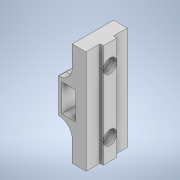
# Autodesk Inventor part: Mount Female
Saved by Autodesk Inventor 2020 (Build 240168000, 168)
## iProperties
Created: 2020-01-14
Part Number: Mount Female
Material: Generic
Document SubType Name: Modeling
Designer: maple
Density: 1 g/cm^3
Appearance: Default
Author: maple
Autodesk Inventor part; units mm, degrees
ref_plane "YZ Plane" through (0, 0, 0) normal (1, 0, 0) x (0, 1, 0)
ref_plane "XZ Plane" through (0, 0, 0) normal (0, 1, 0) x (-1, 0, 0)
ref_plane "XY Plane" through (0, 0, 0) normal (0, 0, 1) x (1, 0, 0)
sketch "Sketch1" plane through (0, 0, 0) normal (0, 1, 0) x (-1, 0, 0)
  line L0 (0, 0) -> (-5.08, 0)
  line L1 (-5.08, 0) -> (-5.08, -15.24)
  line L2 (-5.08, -15.24) -> (0, -15.24)
  line L3 (0, -15.24) -> (0, 0)
  line L4 (-5.08, -7.62) -> (-5.08, -5.08)
  line L5 (-5.08, -5.08) -> (-8.89, -5.08)
  line L6 (-8.89, -5.08) -> (-8.89, -2.54)
  line L7 (-8.89, -5.08) -> (-11.43, -5.08)
  line L8 (-11.43, -5.08) -> (-11.43, -10.16)
  line L9 (-11.43, -10.16) -> (-5.08, -10.16)
  line L10 (-8.89, -10.16) -> (-8.89, -12.7)
  line L11 (-8.89, -12.7) -> (-11.43, -10.16)
  line L12 (-8.89, -2.54) -> (-11.43, -5.08)
  dimension "d0" = 5.08
  dimension "d1" = 15.24
  dimension "d2" = 2.54
  dimension "d3" = 3.81
  dimension "d4" = 2.54
  dimension "d5" = 2.54
  dimension "d6" = 5.08
  dimension "d7" = 2.54
  constraints: 26 end point, 5 perpendicular, 3 point on line, 2 horizontal, 2 parallel, 2 vertical, 1 midpoint
  measures "d0" distance of L2.end L1.end
  measures "d1" distance of L1.end L0.end
  measures "d2" distance of L4.start L4.end
  measures "d3" distance of L4.end L5.end
  measures "d4" distance of L5.end L6.end
  measures "d5" distance of L5.end L7.end
  measures "d6" distance of L7.end L8.end
  measures "d7" distance of L10.start L10.end
extrude "Extrusion1" add sketch "Sketch1" along normal blind 38.1
sketch "Sketch2" plane through (0, 0, -15.24) normal (-1, 0, 0) x (0, 0, 1)
  line L0 (10.16, 0) -> (5.08, 0) projected
  line L1 (7.62, 0) -> (7.62, 7.62)
  line L2 (10.16, 38.1) -> (5.08, 38.1) projected
  line L3 (7.62, 38.1) -> (7.62, 30.48)
  point P0 (15.24, 0)
  dimension "d10" = 7.62
  dimension "d11" = 7.62
  constraints: 4 end point, 2 midpoint, 2 vertical
  measures "d10" distance of L1.start L1.end
  measures "d11" distance of L3.start L3.end
hole "Hole1" at (0, 7.62, -7.62) at (0, 30.48, -7.62) direction (1, 0, 0) diameter 5.08 end through all counterbore diameter 10.16 counterbore depth 3.81
sketch "Sketch3" plane through (0, 0, -15.24) normal (-1, 0, 0) x (0, 0, 1)
  circle A0 centre (7.62, 7.62) radius 5.08 projected
  circle A1 centre (7.62, 30.48) radius 5.08 projected
  line L0 (0, 0) -> (0, 38.1) projected
  line L1 (15.24, 0) -> (15.24, 38.1) projected
  line L2 (0, 12.7) -> (15.24, 12.7)
  line L3 (15.24, 12.7) -> (15.24, 25.4)
  line L4 (15.24, 25.4) -> (0, 25.4)
  line L5 (0, 25.4) -> (0, 12.7)
  dimension "d19" = 12.7
  dimension "d20" = 12.7
  constraints: 8 end point, 2 parallel, 2 point on line, 1 horizontal, 1 perpendicular
  measures "d20" distance of L3.end L2.end
extrude "Extrusion2" add sketch "Sketch3" along normal blind 5.08 contours L2 L0 L4 L1
sketch "Sketch4" plane through (5.08, 0, -15.24) normal (0, 0, -1) x (-1, 0, 0)
  line L0 (10.16, 12.7) -> (10.16, 25.4) projected
  line L1 (10.16, 12.7) -> (8.89, 12.7)
  line L2 (8.89, 12.7) -> (8.89, 13.97)
  line L3 (8.89, 13.97) -> (10.16, 13.97)
  line L4 (10.16, 13.97) -> (10.16, 12.7)
  line L5 (8.89, 13.97) -> (3.81, 13.97)
  line L6 (3.81, 13.97) -> (3.81, 24.13)
  line L7 (3.81, 24.13) -> (8.89, 24.13)
  line L8 (8.89, 24.13) -> (8.89, 13.97)
  point P0 (5.08, 0)
  dimension "d23" = 1.27
  dimension "d24" = 1.27
  dimension "d25" = 5.08
  dimension "d26" = 10.16
  constraints: 16 end point, 4 parallel, 2 horizontal, 2 perpendicular
  measures "d23" distance of L2.end L3.end
  measures "d24" distance of L1.end L2.end
  measures "d25" distance of L6.end L7.end
  measures "d26" distance of L5.end L6.end
extrude "Extrusion3" cut sketch "Sketch4" against normal blind 15.24 contours L5 L6 L7 L8
sketch "Sketch5" plane through (0, 38.1, 0) normal (0, 1, 0) x (1, 0, 0)
  line L0 (0, 0) -> (-5.08, 0) projected
  line L1 (0, 0) -> (6.2992, 0)
  line L2 (6.2992, 0) -> (11.9273, 0)
  line L3 (11.9273, 0) -> (11.9273, 14.1748)
  line L4 (11.9273, 14.1748) -> (6.2992, 14.1748)
  line L5 (6.2992, 14.1748) -> (6.2992, 0)
  dimension "d32" = 6.2992
  constraints: 10 end point, 2 horizontal, 2 parallel, 1 perpendicular
  measures "d32" distance of L0.start L1.end
extrude "Extrusion4" cut sketch "Sketch5" against normal blind 38.1
fillet "Fillet1" radius 4.953 4 edges at (0, 12.7, -3.81) (0, 12.7, -11.43) (0, 25.4, -11.43) (0, 25.4, -3.81)
body "Solid1"
